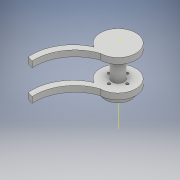
# Autodesk Inventor part: carroussel
Saved by Autodesk Inventor 2017 (Build 210142000, 142)
## iProperties
Part Number: carroussel
Material: Générique
Document SubType Name: Modeling
Designer: Thomas
Density: 1 g/cm^3
Appearance: Par défaut
Author: Thomas
Autodesk Inventor part; units mm, degrees
ref_plane "YZ Plane" through (0, 0, 0) normal (1, 0, 0) x (0, 1, 0)
ref_plane "XZ Plane" through (0, 0, 0) normal (0, 1, 0) x (-1, 0, 0)
ref_plane "XY Plane" through (0, 0, 0) normal (0, 0, 1) x (1, 0, 0)
sketch "Esquisse1" plane through (0, 0, 0) normal (0, 0, 1) x (1, 0, 0)
  circle A0 centre (0, 0) radius 1.35
  circle A1 centre (0, -7.75) radius 1.15
  circle A2 centre (7.75, 0) radius 1.15
  circle A3 centre (0, 7.75) radius 1.15
  circle A4 centre (-7.75, 0) radius 1.15
  circle A5 centre (0, 0) radius 11
  constraints: 6 centre point
extrude "Extrusion1" add sketch "Esquisse1" along normal blind 10
sketch "Esquisse3" plane through (0, 0, 10) normal (0, 0, 1) x (1, 0, 0)
  circle A0 centre (0, 0) radius 1.35 projected
  arc A1 (0, -15) -> (-7.3469, -13.0776) centre (0, 0) ccw
  arc A2 (-7.3469, -13.0776) -> (-27.8845, -48.1677) centre (6.8982, -44.9701) ccw
  arc A3 (0, -15) -> (-23.2475, -49.4967) centre (11.2565, -47.6674) ccw
  line L0 (-27.8845, -48.1677) -> (-23.2475, -49.4967)
  dimension "d28" = 30
  constraints: 6 point on circle, 3 centre point, 2 end point, 1 coincident
  measures "d28" diameter of A1
extrude "Extrusion3" add sketch "Esquisse3" along normal blind 5
sketch "Esquisse4" plane through (0, 0, 0) normal (0, 0, -1) x (-1, 0, 0)
  circle A0 centre (0, 0) radius 1.35 projected
  circle A1 centre (7.75, 0) radius 1.15 projected
  circle A2 centre (0, 7.75) radius 1.15 projected
  circle A3 centre (-7.75, 0) radius 1.15 projected
  circle A4 centre (0, -7.75) radius 1.15 projected
  circle A5 centre (0, 0) radius 11 projected
extrude "Extrusion4" cut sketch "Esquisse4" against normal blind 46.25 contours A0 | A1 | A2 | A3 | A4
sketch "Esquisse5" plane through (0, 0, 15) normal (0, 0, 1) x (1, 0, 0)
  circle A0 centre (0, 0) radius 5
  dimension "d33" = 10
  constraints: 1 centre point, 1 coincident
  measures "d33" diameter of A0
extrude "Extrusion5" add sketch "Esquisse5" along normal blind 26
pattern_linear "Réseau rectangulaire1" count 2 spacing 26 along (0, 0, 1) of "Extrusion3"
sketch "Esquisse6" plane through (0, 0, 0) normal (0, 0, -1) x (-1, 0, 0)
  circle A0 centre (0, 0) radius 1.35 projected
  circle A1 centre (0, 0) radius 11
  constraints: 1 centre point, 1 coincident
extrude "Extrusion6" cut sketch "Esquisse6" against normal blind 5
